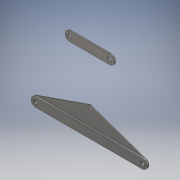
# Autodesk Inventor part: Cabin Hold
Saved by Autodesk Inventor 2019 (Build 230136000, 136)
## iProperties
Created: 2019-08-30
Part Number: Cabin Hold
Material: Steel, Mild
Document SubType Name: Modeling
Designer: DIBYOJYOTI
Density: 7.85 g/cm^3
Appearance: Semi-Polished
Author: DIBYOJYOTI
Autodesk Inventor part; units mm, degrees
ref_plane "YZ Plane" through (0, 0, 0) normal (1, 0, 0) x (0, 1, 0)
ref_plane "XZ Plane" through (0, 0, 0) normal (0, 1, 0) x (-1, 0, 0)
ref_plane "XY Plane" through (0, 0, 0) normal (0, 0, 1) x (1, 0, 0)
derived "Cabin Wall.ipt"
sketch "Sketch2" plane through (0, 0, 0) normal (0, 0, 1) x (1, 0, 0)
  circle A0 centre (80, 30) radius 2.05
  circle A1 centre (50, 110) radius 3
  circle A2 centre (110, 110) radius 3
  circle A3 centre (160, 0) radius 3
  circle A4 centre (0, 0) radius 3
  line L0 (50, 110) -> (110, 110) construction
  line L1 (50, 103) -> (110, 103)
  line L2 (110, 117) -> (50, 117)
  arc A5 (50, 117) -> (50, 103) centre (50, 110) ccw
  arc A6 (110, 103) -> (110, 117) centre (110, 110) ccw
  line L3 (160, 0) -> (157, 0) construction
  line L4 (3, 0) -> (0, 0) construction
  line L5 (0, 0) -> (160, 0) construction
  line L6 (0, -7) -> (160, -7)
  line L7 (160, 7) -> (0, 7)
  arc A7 (0, 7) -> (0, -7) centre (0, 0) ccw
  arc A8 (160, -7) -> (160, 7) centre (160, 0) ccw
  arc A9 (81.6455, 34.7215) -> (78.3545, 34.7215) centre (80, 30) ccw
  line L8 (-2.3038, 6.61) -> (78.3545, 34.7215)
  line L9 (162.3038, 6.61) -> (81.6455, 34.7215)
  point P0 (80, 110)
  point P1 (80, 0)
  dimension "d16" = 6
  dimension "d17" = 6
  dimension "d9" = 60
  dimension "d10" = 7
  dimension "d11" = 6
  dimension "d12" = 4.1
  dimension "d13" = 5
  dimension "d14" = 160
  dimension "d15" = 14
  dimension "d18" = 30
  constraints: 20 end point, 10 point on circle, 8 centre point, 2 horizontal alignment, 2 other
  measures "d9" distance of L0.end A1.centre
  measures "d10" radius of A6
  measures "d11" diameter of A2
  measures "d12" diameter of A0
  measures "d13" radius of A9
  measures "d14" distance of point (0, 0) L3.start
  measures "d15" distance between parallel lines of L6 L7
  measures "d18" distance of point (80, 0) A9.centre
extrude "Extrusion1" add sketch "Sketch2" along normal blind 2 and the other way blind 1 contours A7 L7 A8 L6
extrude "Extrusion2" add sketch "Sketch2" along normal mid plane 2 contours A5 L2 A6 L1
extrude "Extrusion3" add sketch "Sketch2" against normal blind 1 contours L8 A9 L9 A8 L7 A7
body "Solid1"
